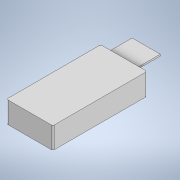
# Autodesk Inventor part: Modulo NRF24 2
Saved by Autodesk Inventor 2021.4 (Build 254397000, 397)
## iProperties
Created: 2022-11-18
Part Number: Modulo NRF24 2
Material: Genérico
Document SubType Name: Modeling
Designer: crist
Density: 1 g/cm^3
Appearance: Valor por defecto
Author: crist
Autodesk Inventor part; units mm, degrees
ref_plane "YZ Plane" through (0, 0, 0) normal (1, 0, 0) x (0, 1, 0)
ref_plane "XZ Plane" through (0, 0, 0) normal (0, 1, 0) x (-1, 0, 0)
ref_plane "XY Plane" through (0, 0, 0) normal (0, 0, 1) x (1, 0, 0)
sketch "Boceto1" plane through (0, 0, 0) normal (0, 1, 0) x (-1, 0, 0)
  line L0 (1, 0) -> (27, 0)
  line L1 (28, -1) -> (28, -56)
  line L2 (27, -57) -> (1, -57)
  line L3 (0, -56) -> (0, -1)
  arc A0 (28, -1) -> (27, 0) centre (27, -1) ccw
  arc A1 (27, -57) -> (28, -56) centre (27, -56) ccw
  arc A2 (0, -56) -> (1, -57) centre (1, -56) ccw
  arc A3 (1, 0) -> (0, -1) centre (1, -1) ccw
  point P0 (0, 0)
  point P1 (28, -57)
  point P2 (28, 0)
  point P3 (0, -57)
  dimension "d0" = 57
  dimension "d1" = 28
  dimension "d2" = 1
  constraints: 8 end point, 8 point on circle, 8 point on line, 8 tangent, 4 centre point, 3 equal radius, 2 parallel, 1 horizontal, 1 perpendicular
  measures "d0" distance of point (28, 0) point (28, -57)
  measures "d1" distance of point (28, -57) point (0, -57)
  measures "d2" radius of A0
extrude "Extrusión1" add sketch "Boceto1" along normal blind 13
sketch "Boceto2" plane through (-1, 0, -57) normal (0, 0, -1) x (-1, 0, 0)
  line L0 (-1, 0) -> (-1, 13)
  line L1 (-1, 13) -> (7, 13)
  line L2 (7, 10) -> (7, 9)
  line L3 (7, 9) -> (24, 9)
  line L4 (24, 9) -> (24, 10)
  line L5 (7, 10) -> (24, 10)
  line L6 (26, 13) -> (0, 13) projected
  line L7 (7, 13) -> (7, 10)
  dimension "d5" = 8
  dimension "d6" = 1
  dimension "d7" = 17
  dimension "d11" = 3
  constraints: 14 end point, 5 perpendicular, 1 vertical
  measures "d5" distance of L1.end L0.end
  measures "d6" distance of L2.start L2.end
  measures "d7" distance of L2.end L3.end
  measures "d11" distance of L1.end L7.end
extrude "Extrusión2" add sketch "Boceto2" along normal blind 16
